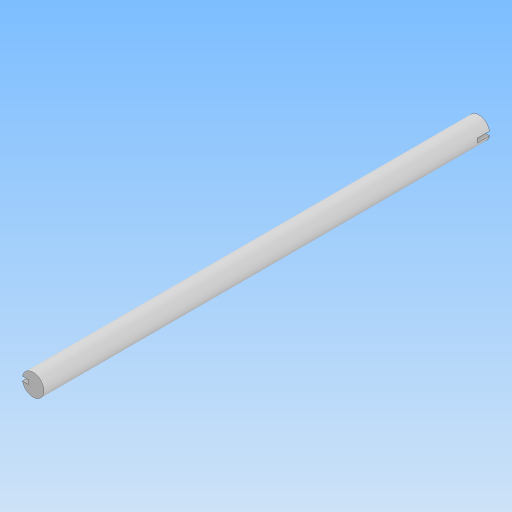
# Autodesk Inventor part: Welle
Saved by Autodesk Inventor 2024.4 (Build 284460000, 460)
## iProperties
Created: 2026-01-19
Part Number: Welle
Material: Generisch
Document SubType Name: Modeling
Designer: windows-desktop
Density: 1 g/cm^3
Appearance: Vorgabe
Mass: 694.266 g
Surface Area: 823.416 cm^2
Volume: 694.266 cm^3
Masse[kg]: 0,694 kg
Author: windows-desktop
Autodesk Inventor part; units mm, degrees
ref_plane "XZ Plane" through (0, 0, 0) normal (0, 1, 0) x (-1, 0, 0)
sketch "Skizze1" plane through (0, 0, 0) normal (0, 1, 0) x (-1, 0, 0)
  circle A0 centre (0, 0) radius 17.5
  dimension "d0" = 35
  constraints: 1 centre point, 1 coincident
  measures "d0" diameter of A0
extrude "Extrusion1" add sketch "Skizze1" along normal blind 724.33
ref_plane "Arbeitsebene1" through (-7.5, 0, 0) normal (1, 0, 0) x (0, 1, 0)
sketch "Skizze2" plane through (-7.5, 0, 0) normal (1, 0, 0) x (0, 1, 0)
  line L0 (0, 0) -> (0, 3.311)
  line L1 (0, -17.5) -> (0, 17.5) construction
  line L2 (0, 0) -> (0, -3.311)
  line L3 (0, 3.311) -> (20, 3.311)
  line L4 (20, 3.311) -> (20, -3.311)
  line L5 (20, -3.311) -> (0, -3.311)
  line L6 (0, -3.311) -> (0, 3.311)
  dimension "d4" = 3.311
  dimension "d5" = 3.311
  dimension "d6" = 20
  constraints: 12 end point, 2 parallel, 2 point on line, 1 horizontal, 1 perpendicular
  measures "d4" distance of L0.start L0.end
  measures "d5" distance of L0.start L2.end
  measures "d6" distance of L4.end L5.end
extrude "Extrusion2" cut sketch "Skizze2" against normal blind 724.33
ref_plane "Arbeitsebene2" through (7.5, 0, 0) normal (1, 0, 0) x (0, 1, 0)
sketch "Skizze3" plane through (7.5, 0, 0) normal (1, 0, 0) x (0, 1, 0)
  line L0 (724.33, -17.5) -> (724.33, 17.5) construction
  line L1 (724.33, 0) -> (724.33, 3.311)
  line L2 (724.33, 0) -> (724.33, -3.311)
  line L3 (724.33, 3.311) -> (704.33, 3.311)
  line L4 (704.33, 3.311) -> (704.33, -3.311)
  line L5 (704.33, -3.311) -> (724.33, -3.311)
  line L6 (724.33, -3.311) -> (724.33, 3.311)
  point P0 (0, 0)
  dimension "d10" = 3.311
  dimension "d11" = 3.311
  dimension "d12" = 20
  constraints: 12 end point, 2 parallel, 2 point on line, 1 horizontal, 1 midpoint, 1 perpendicular
  measures "d10" distance of L1.start L1.end
  measures "d11" distance of L1.start L2.end
  measures "d12" distance of L5.end L4.end
extrude "Extrusion3" cut sketch "Skizze3" along normal blind 724.33
equation "\"d0\" = Wellensdurchmesser"
equation "\"d1\" = Wellenlänge"
equation "\"d7\" = Wellenlänge"
equation "\"d13\" = Wellenlänge"
equation "\"Wellensdurchmesser\" = 35"
equation "\"Wellenlänge\" = 724.33"
